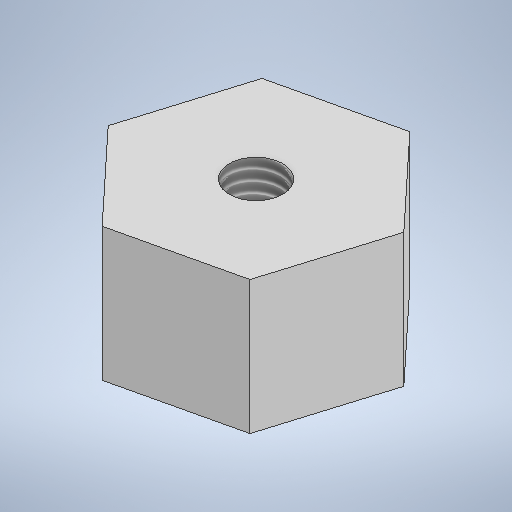
# Autodesk Inventor part: nakretka_m2
Saved by Autodesk Inventor 2025.2 (Build 292293000, 293)
## iProperties
Created: 2025-11-27
Part Number: nakretka_m2
Material: Ogólny
Document SubType Name: Modeling
Designer: juras
Density: 1 g/cm^3
Appearance: Domyślna
Author: juras
Autodesk Inventor part; units mm, degrees
ref_plane "YZ Plane" through (0, 0, 0) normal (1, 0, 0) x (0, 1, 0)
ref_plane "XZ Plane" through (0, 0, 0) normal (0, 1, 0) x (-1, 0, 0)
ref_plane "XY Plane" through (0, 0, 0) normal (0, 0, 1) x (1, 0, 0)
sketch "Szkic1" plane through (0, 0, 0) normal (0, 1, 0) x (-1, 0, 0)
  line L0 (-1.3486, -4.4175) -> (-4.5, -1.0408)
  line L1 (-4.5, -1.0408) -> (-3.1514, 3.3767)
  line L2 (-3.1514, 3.3767) -> (1.3486, 4.4175)
  line L3 (1.3486, 4.4175) -> (4.5, 1.0408)
  line L4 (4.5, 1.0408) -> (3.1514, -3.3767)
  line L5 (3.1514, -3.3767) -> (-1.3486, -4.4175)
  point P0 (0, 0)
  point P1 (0, 0)
  dimension "d0" = 4
  dimension "d1" = 4.5
  constraints: 12 end point, 1 coincident, 13 other
  measures "d0" distance from line of L5 point (0, 0)
  measures "d1" horizontal distance of L4.end L0.start
extrude "Wyciągnięcie proste1" add sketch "Szkic1" along normal blind 5
sketch "Szkic2" plane through (0, 5, 0) normal (0, 1, 0) x (1, 0, 0)
  circle A0 centre (0, 0) radius 1
  dimension "d4" = 2
  constraints: 1 centre point, 1 coincident
  measures "d4" diameter of A0
extrude "Wyciągnięcie proste2" cut sketch "Szkic2" against normal blind 5
thread "Gwint1" size "M2x0.4" class "6H" standard "ANSI Metric M Profile" length 25
